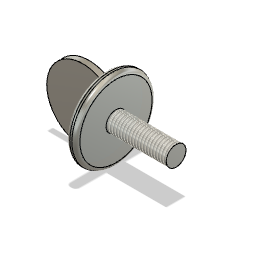
Pin v1 (Autodesk Fusion 360 design; units mm, degrees)
Autodesk Fusion 360 part; units mm, degrees
sketch "Sketch1" plane through (0, 0, 0) normal (1, 0, 0) x (0, 0, -1)
  circle A0 centre (-25, 15) radius 20
  dimension "d1" = 40
  measures "d1" diameter of A0
extrude "Extrude1" add sketch "Sketch1" along normal blind 5
fillet "Fillet1" radius 2 1 edges at (5, 7.7677, 43.6465)
fillet "Fillet2" radius 2 1 edges at (0, 7.7677, 43.6465)
sketch "Sketch2" plane through (5, 0, 0) normal (1, 0, 0) x (0, 0, -1)
  circle A0 centre (-25, 15) radius 18
  circle A1 centre (-25, 15) radius 5
  dimension "d6" = 10
  constraint concentric A0 A1
  measures "d6" diameter of A1
extrude "Extrude2" add sketch "Sketch2" along normal blind 30 contours A1
thread "Thread1" "ISO Metric profile 10.0 M10x1.5 6g" major diameter 9.85 minor diameter 8.141 pitch 1.5 angle 60 resizes the face on face at (25, 14.5022, 20.0248)
sketch "Sketch3" plane through (0, 0, 0) normal (1, 0, 0) x (0, 0, -1)
sketch "Sketch4" plane through (0, 0, 0) normal (-1, 0, 0) x (0, 0, 1)
  circle A0 centre (25, 15) radius 18
sketch "Sketch5" plane through (0, 0, 0) normal (0, 0, 1) x (1, 0, 0)
sketch "Sketch6" plane through (0, 0, 0) normal (0, 0, 1) x (1, 0, 0)
  line L0 (-10, 15) -> (50, 15)
  line L1 (0, 0) -> (0, 29.9666)
  arc A0 (0, 29.9666) -> (0, 0.0334) centre (-10, 15) ccw
  dimension "d9" = 36
  constraint coincident L0.start A0.centre
  constraint coincident L1.start origin
  constraint vertical L1
  constraint coincident L1 A0.end
  measures "d9" diameter of A0
extrude "Extrude3" add sketch "Sketch6" along normal blind 3 from surface at 23.5
